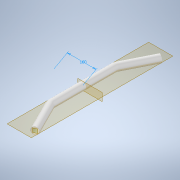
# Autodesk Inventor part: caña bici ruta
Saved by Autodesk Inventor 2021 (Build 250183000, 183)
## iProperties
Created: 2021-07-10
Part Number: caña bici ruta
Material: Generic
Document SubType Name: Modeling
Designer: j2seb
Density: 1 g/cm^3
Appearance: Default
Author: j2seb
Autodesk Inventor part; units mm, degrees
ref_plane "YZ Plane" through (0, 0, 0) normal (1, 0, 0) x (0, 1, 0)
ref_plane "XZ Plane" through (0, 0, 0) normal (0, 1, 0) x (-1, 0, 0)
ref_plane "XY Plane" through (0, 0, 0) normal (0, 0, 1) x (1, 0, 0)
sketch "Sketch1" plane through (0, 0, 0) normal (0, 1, 0) x (-1, 0, 0)
  line L0 (-95.7003, 304.5005) -> (-5.7003, 154.5005)
  line L1 (0, 133.9206) -> (0, 0)
  line L2 (53.8545, 0) -> (-53.8545, 0)
  line L3 (-95.7003, -304.5005) -> (-5.7003, -154.5005)
  line L4 (0, -133.9206) -> (0, 0)
  arc A0 (0, 133.9206) -> (-5.7003, 154.5005) centre (-40, 133.9206) ccw
  arc A1 (-5.7003, -154.5005) -> (0, -133.9206) centre (-40, -133.9206) ccw
  point P0 (0, 145)
  point P1 (0, -145)
  dimension "d0" = 145
  dimension "d1" = 40
  dimension "d2" = 90
  dimension "d3" = 150
  dimension "d8" = 40
  constraints: 10 end point, 4 point on circle, 4 point on line, 4 tangent, 2 centre point, 2 symmetric about line, 1 horizontal, 1 midpoint, 1 vertical
  measures "d0" distance of point (0, 145) L1.end
  measures "d1" radius of A0
  measures "d2" horizontal distance of L0.end L0.start
  measures "d3" vertical distance of L0.start L0.end
  measures "d8" radius of A1
ref_plane "Work Plane1" through (95.7003, 0, 304.5005) normal (-0.5145, 0, -0.8575) x (0, -1, 0)
sketch "Sketch2" plane through (95.7003, 0, 304.5005) normal (-0.5145, 0, -0.8575) x (0, -1, 0)
  circle A0 centre (0, 0) radius 20
  circle A1 centre (0, 0) radius 18.5
  point P0 (0, -74.6019)
  dimension "d4" = 40
  dimension "d5" = 37
  constraints: 2 centre point, 1 coincident
  measures "d4" diameter of A0
  measures "d5" diameter of A1
sweep "Sweep1" add profiles "Sketch2" path "Sketch1" path curves L0 A0 L1 L4 A1 L3
equation "\"d8\" = d1"
body "Solid1"
